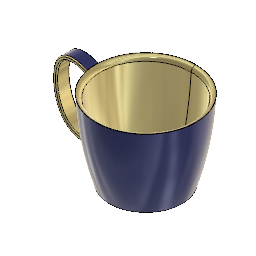
kubek złoty v2 (Autodesk Fusion 360 design; units mm, degrees)
Autodesk Fusion 360 part; units mm, degrees
sketch "Sketch1" plane through (0, 0, 0) normal (1, 0, 0) x (0, 1, 0)
  line L0 (0, 170) -> (0, 0)
  line L1 (0, 0) -> (80, 0)
  spline S0 degree 5 poles (80, 0) (81.0088, 3.1678) (82.9904, 9.524) (85.8544, 19.1198) (89.453, 32.0391) (93.5599, 48.4105) (97.2417, 65.0233) (100.4659, 81.896) (103.2186, 99.0364) (105.5226, 116.4317) (107.4136, 134.0614) (108.6242, 148.3369) (109.3729, 159.1339) (109.8026, 166.3714) (110, 170) knots 0 0 0 0 0 0 0.1 0.2 0.3 0.4 0.5 0.6 0.7 0.8 0.9 1 1 1 1 1 1
  line L2 (0, 170) -> (110, 170)
  point P0 (100, 80)
  constraint coincident L0.end L1.start
  constraint vertical L0
  constraint perpendicular L0 L1
  constraint perpendicular L0 L2
revolve "Revolve1" add sketch "Sketch1" angle 360 about axis through (0, 0, 170) along (0, 0, -1)
shell "Shell1" thickness 10 removed faces 1 at (5.5282, -19.6526, 170)
fillet "Fillet1" radius 10 1 edges at (0.0456, -99.985, 170)
sketch "Sketch2" plane through (0, 0, 0) normal (0, 1, 0) x (1, 0, 0)
  spline S0 degree 5 poles (-103.0556, -154.9451) (-108.0216, -157.3937) (-117.6034, -161.7232) (-130.9261, -166.5143) (-146.574, -169.4717) (-162.5186, -167.3927) (-174.7421, -159.6354) (-183.1605, -146.5981) (-187.7726, -129.2011) (-188.6906, -108.961) (-186.0842, -87.6926) (-180.1553, -67.3042) (-171.1141, -49.5635) (-159.1671, -35.8782) (-144.5111, -27.0407) (-127.3149, -23.402) (-111.6275, -24.7117) (-98.8111, -28.0436) (-89.8032, -31.3016) (-85.1833, -33.1897) knots 0 0 0 0 0 0 0.066667 0.133333 0.2 0.266667 0.333333 0.4 0.466667 0.533333 0.6 0.666667 0.733333 0.8 0.866667 0.933333 1 1 1 1 1 1
  point P0 (-180, -150)
  point P1 (-170, -50)
ref_plane "WorkPlane1" through (-109.0626, 0, 155.038) normal (-0.997488, 0, -0.070842) x (0, -1, 0)
sketch "Sketch3" plane through (-109.0626, 0, 155.038) normal (-0.997488, 0, -0.070842) x (0, -1, 0)
  line L0 (-12.5, 5) -> (12.5, 5)
  line L1 (15, 2.5) -> (15, -2.5)
  line L2 (12.5, -5) -> (-12.5, -5)
  line L3 (-15, -2.5) -> (-15, 2.5)
  arc A0 (-12.5, 5) -> (-15, 2.5) centre (-12.5, 2.5) ccw
  arc A1 (15, 2.5) -> (12.5, 5) centre (12.5, 2.5) ccw
  arc A2 (12.5, -5) -> (15, -2.5) centre (12.5, -2.5) ccw
  arc A3 (-15, -2.5) -> (-12.5, -5) centre (-12.5, -2.5) ccw
  dimension "d5" = 2.5
  constraint horizontal L0
  constraint vertical L1
  constraint horizontal L2
  constraint vertical L3
  constraint tangent L0 A0
  constraint tangent L3 A0
  constraint tangent L0 A1
  constraint tangent L1 A1
  constraint equal A0 A1
  constraint tangent L1 A2
  constraint tangent L2 A2
  constraint equal A0 A2
  constraint tangent L2 A3
  constraint tangent L3 A3
  constraint equal A0 A3
  measures "d5" radius of A0
sweep "Sweep1" add profiles "Sketch3" path "Sketch2" along S0 section 1
